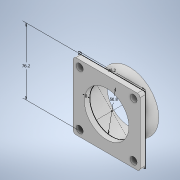
# Autodesk Inventor part: chumacera
Saved by Autodesk Inventor 2021 (Build 250183000, 183)
## iProperties
Created: 2022-02-18
Part Number: chumacera
Material: Genérico
Document SubType Name: Modeling
Designer: arthu
Density: 1 g/cm^3
Appearance: Valor por defecto
Author: arthu
Autodesk Inventor part; units mm, degrees
ref_plane "YZ Plane" through (0, 0, 0) normal (1, 0, 0) x (0, 1, 0)
ref_plane "XZ Plane" through (0, 0, 0) normal (0, 1, 0) x (-1, 0, 0)
ref_plane "XY Plane" through (0, 0, 0) normal (0, 0, 1) x (1, 0, 0)
sketch "Boceto1" plane through (0, 0, 0) normal (0, 0, 1) x (1, 0, 0)
  line L0 (38.1, -38.1) -> (-38.1, -38.1)
  line L1 (-38.1, -38.1) -> (-38.1, 38.1)
  line L2 (-38.1, 38.1) -> (38.1, 38.1)
  line L3 (38.1, 38.1) -> (38.1, -38.1)
  line L4 (38.1, -38.1) -> (-38.1, 38.1) construction
  line L5 (-38.1, -38.1) -> (38.1, 38.1) construction
  circle A0 centre (0, 0) radius 25.4
  circle A1 centre (0, 0) radius 33.4
  dimension "d0" = 76.2
  dimension "d1" = 76.2
  dimension "d2" = 50.8
  dimension "d3" = 8
  constraints: 12 end point, 2 centre point, 2 midpoint, 2 parallel, 1 coincident, 1 horizontal, 1 perpendicular
  measures "d0" distance of L1.end L2.end
  measures "d1" distance between parallel lines of L0 L2
  measures "d2" diameter of A0
  measures "d3" radial gap between concentric circles of A0 A1
extrude "Extrusión1" add sketch "Boceto1" along normal blind 6 contours L0 L1 L2 L3 | A1
extrude "Extrusión2" add sketch "Boceto1" against normal blind 20 contours A1
sketch "Boceto2" plane through (0, 0, 0) normal (0, 0, -1) x (-1, 0, 0)
  line L0 (-38.1, 38.1) -> (38.1, 38.1) projected
  circle A0 centre (0, 0) radius 25.4 projected
  line L1 (38.1, 38.1) -> (38.1, -38.1) projected
  line L2 (38.1, -38.1) -> (-38.1, -38.1) projected
  line L3 (-38.1, -38.1) -> (-38.1, 38.1) projected
  circle A1 centre (30.7591, 30.7591) radius 4
  circle A2 centre (-30.7591, 30.7591) radius 4
  circle A3 centre (-30.7591, -30.7591) radius 4
  circle A4 centre (30.7591, -30.7591) radius 4
  dimension "d10" = 8
  dimension "d11" = 8
  dimension "d12" = 8
  dimension "d13" = 8
  constraints: 4 centre point
  measures "d10" diameter of A1
  measures "d11" diameter of A2
  measures "d12" diameter of A3
  measures "d13" diameter of A4
extrude "Extrusión3" cut sketch "Boceto2" against normal blind 20 contours A1 | A2 | A3 | A4
fillet "Empalme1" radius 3 4 edges at (-38.1, 38.1, 3) (38.1, 38.1, 3) (38.1, -38.1, 3) (-38.1, -38.1, 3)
